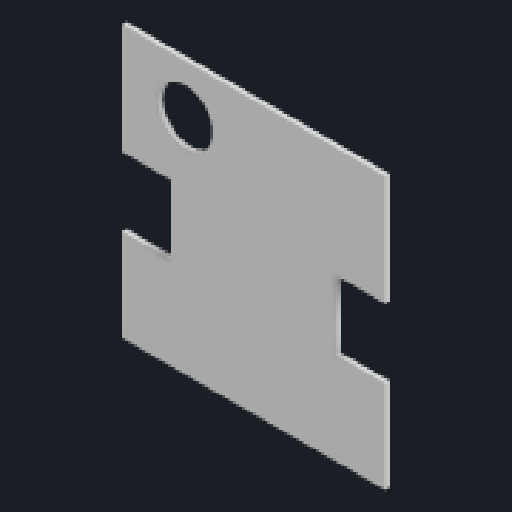
# Autodesk Inventor part: ФАЛЬШБОРТА 2
Saved by Autodesk Inventor 2025 (Build 290162000, 162)
## iProperties
Created: 2025-01-26
Part Number: ФАЛЬШБОРТА 2
Material: Типовые
Document SubType Name: Modeling
Designer: GameHD
Density: 1 g/cm^3
Appearance: По умолчанию
Author: GameHD
Autodesk Inventor part; units mm, degrees
ref_plane "YZ Plane" through (0, 0, 0) normal (1, 0, 0) x (0, 1, 0)
ref_plane "XZ Plane" through (0, 0, 0) normal (0, 1, 0) x (-1, 0, 0)
ref_plane "XY Plane" through (0, 0, 0) normal (0, 0, 1) x (1, 0, 0)
sketch "Эскиз1" plane through (0, 0, 0) normal (0, 0, 1) x (1, 0, 0)
  line L0 (0, 0) -> (230, 0)
  line L1 (230, 0) -> (230, 238)
  line L2 (230, 238) -> (0, 238)
  line L3 (0, 238) -> (0, 0)
  dimension "d0" = 230
  dimension "d1" = 238
  constraints: 8 end point, 2 parallel, 1 horizontal, 1 perpendicular
  measures "d0" distance of L2.end L1.end
  measures "d1" distance of L1.end L0.end
extrude "Выдавливание1" add sketch "Эскиз1" along normal blind 4
sketch "Эскиз2" plane through (0, 0, 0) normal (0, 0, -1) x (-1, 0, 0)
  arc A0 (-51.7131, 177.8967) -> (-37.5771, 193.5505) centre (-55.4712, 195.5) ccw projected
  circle A1 centre (-55.4712, 195.5) radius 23.7641
  line L0 (-234.95, 80.9625) -> (-187.325, 80.9625)
  line L1 (-187.325, 80.9625) -> (-187.325, 141.2875)
  line L2 (-187.325, 141.2875) -> (-234.95, 141.2875)
  line L3 (-234.95, 141.2875) -> (-234.95, 80.9625)
  line L4 (-234.95, 80.9625) -> (-187.325, 141.2875) construction
  line L5 (-187.325, 80.9625) -> (-234.95, 141.2875) construction
  line L6 (-230, 238) -> (0, 238) projected
  line L7 (-115, 238) -> (-115, 103.1875)
  line L8 (4.95, 80.9625) -> (-42.675, 80.9625)
  line L9 (-42.675, 80.9625) -> (-42.675, 141.2875)
  line L10 (-42.675, 141.2875) -> (4.95, 141.2875)
  line L11 (4.95, 141.2875) -> (4.95, 80.9625)
  line L12 (4.95, 80.9625) -> (-42.675, 141.2875) construction
  line L13 (-42.675, 80.9625) -> (4.95, 141.2875) construction
  point P0 (0, 0)
  point P1 (-211.1375, 111.125)
  point P2 (-18.8625, 111.125)
  constraints: 26 end point, 5 symmetric about line, 3 midpoint, 2 parallel, 1 centre point, 1 coincident, 1 horizontal, 1 perpendicular, 1 vertical
extrude "Выдавливание2" cut sketch "Эскиз2" against normal blind 4
